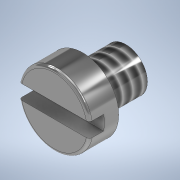
# Autodesk Inventor part: Peça10
Saved by Autodesk Inventor 2021 (Build 250183000, 183)
## iProperties
Created: 2020-11-15
Part Number: Peça10
Material: Liga de Nickel-Copper 400
Document SubType Name: Modeling
Designer: Bruno
Density: 8.83 g/cm^3
Appearance: Cromado - Preto polido
Author: Bruno
Autodesk Inventor part; units mm, degrees
ref_plane "YZ Plane" through (0, 0, 0) normal (1, 0, 0) x (0, 1, 0)
ref_plane "XZ Plane" through (0, 0, 0) normal (0, 1, 0) x (-1, 0, 0)
ref_plane "XY Plane" through (0, 0, 0) normal (0, 0, 1) x (1, 0, 0)
sketch "Esboço1" plane through (0, 0, 0) normal (0, 0, 1) x (1, 0, 0)
  circle A0 centre (0, 0) radius 1.25
  dimension "d0" = 2.5
  constraints: 1 centre point, 1 coincident
  measures "d0" diameter of A0
extrude "Extrusão1" add sketch "Esboço1" along normal blind 1
sketch "Esboço2" plane through (0, 0, 0) normal (0, 0, -1) x (-1, 0, 0)
  circle A0 centre (0, 0) radius 0.75
  dimension "d3" = 1.5
  constraints: 1 centre point, 1 coincident
  measures "d3" diameter of A0
extrude "Extrusão2" add sketch "Esboço2" along normal blind 1.5
sketch "Esboço3" plane through (0, 0, 1) normal (0, 0, 1) x (1, 0, 0)
  circle A0 centre (0, 0) radius 1.25 projected
  line L0 (-1.2241, -0.2529) -> (1.2241, -0.2529)
  line L1 (1.2241, -0.2529) -> (1.2241, 0.2529)
  line L2 (1.2241, 0.2529) -> (-1.2241, 0.2529)
  line L3 (-1.2241, 0.2529) -> (-1.2241, -0.2529)
  line L4 (-1.2241, -0.2529) -> (1.2241, 0.2529) construction
  line L5 (1.2241, -0.2529) -> (-1.2241, 0.2529) construction
  dimension "d6" = 2.4483
  constraints: 12 end point, 2 midpoint, 2 parallel, 1 horizontal, 1 perpendicular, 1 point on circle
  measures "d6" distance of L0.start L0.end
extrude "Extrusão3" cut sketch "Esboço3" against normal blind 0.5 contours L1 L0 L3 L2
sketch "Esboço4" plane through (-1.2241, -0.2529, 1) normal (1, 0, 0) x (0, 0, -1)
  line L0 (0, 0.5058) -> (0, 0) projected
  line L1 (0.5, 0) -> (0.5, 0.5058) projected
  line L2 (0, 0.5058) -> (0.5, 0.5058)
  line L3 (0.5, 0.5058) -> (0.5, 0)
  line L4 (0.5, 0) -> (0, 0) projected
  line L5 (0.5, 0) -> (0, 0)
  line L6 (0, 0) -> (0, 0.5058)
  point P0 (1, 0.2529)
  constraints: 8 end point, 3 perpendicular, 1 collinear
extrude "Extrusão4" cut sketch "Esboço4" along normal mid plane 6
fillet "Arredondamento1" radius 0.1 1 edges at (0, 1.25, 1)
fillet "Arredondamento1" radius 0.1 1 edges at (0, -1.25, 1)
thread "Rosca1" size "M1.6x0.35" class "6g" standard "ANSI Metric M Profile" length 15.255
